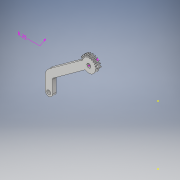
# Autodesk Inventor part: sem2_thumb-finger2
Saved by Autodesk Inventor 2018 (Build 220112000, 112)
## iProperties
Created: 2017-10-02
Part Number: sem2_thumb-finger2
Material: Generic
Document SubType Name: Modeling
Designer: rheal
Density: 1 g/cm^3
Appearance: Default
Author: rheal
Autodesk Inventor part; units mm, degrees
note: some values were not read from the file. Chosen so that the rebuilt part matches the saved one: pattern direction of "Circular Pattern2".
ref_plane "YZ Plane" through (0, 0, 0) normal (1, 0, 0) x (0, 1, 0)
ref_plane "XZ Plane" through (0, 0, 0) normal (0, 1, 0) x (-1, 0, 0)
ref_plane "XY Plane" through (0, 0, 0) normal (0, 0, 1) x (1, 0, 0)
sketch "Sketch1" plane through (0, 0, 0) normal (0, 0, 1) x (1, 0, 0)
  arc A0 (-83.5272, 11.9642) -> (-77.9867, 11.6439) centre (-80.7477, 11.9642) ccw
  line L0 (-50.0146, 32.1007) -> (-50.0146, 50.0136) construction
  arc A1 (-52.8662, 40.9092) -> (-54.8238, 46.3734) centre (-50.0146, 45.0136) ccw
  line L1 (-83.5272, 11.9642) -> (-83.5272, 22.4192)
  arc A2 (-83.5272, 11.9642) -> (-77.9681, 11.9642) centre (-80.7477, 11.9642) ccw
  line L2 (-77.9681, 11.9642) -> (-77.9681, 21.7768)
  line L3 (-52.8662, 40.9092) -> (-77.1364, 23.2751)
  line L4 (-80.4111, 27.7823) -> (-56.141, 45.4163)
  arc A3 (-80.4111, 27.7823) -> (-83.5272, 22.4192) centre (-76.1194, 21.702) ccw
  arc A4 (-77.1364, 23.2751) -> (-77.9681, 21.7768) centre (-76.2028, 21.7768) ccw
  line L5 (-52.8662, 40.9092) -> (-56.141, 45.4163)
  line L6 (-77.1364, 23.2751) -> (-80.4111, 27.7823)
  line L7 (-56.141, 45.4163) -> (-54.8238, 46.3734)
  arc A5 (-54.7992, 43.5696) -> (-54.8238, 46.3734) centre (-50.0146, 45.0136) ccw
  line L8 (-52.8662, 40.9092) -> (-77.1364, 23.2751)
  line L9 (-77.1364, 23.2751) -> (-80.4111, 27.7823)
  point P0 (19.05, 139.7)
  point P1 (-45.0223, 44.7358)
  point P2 (-77.9681, 22.6804)
  dimension "d69" = 2.7795
  dimension "d107" = 30
  constraints: 20 end point, 13 point on circle, 6 centre point, 2 perpendicular, 2 point on line, 2 tangent, 2 vertical, 1 coincident, 1 collinear, 1 concentric, 1 parallel
  measures "d69" radius of A0
  measures "d107" distance of L3.end L3.start
extrude "Extrusion1" add sketch "Sketch1" along normal blind 3
sketch "Sketch15" plane through (0, 0, 0) normal (0, 0, -1) x (-1, 0, 0)
  point P0 (0, 0)
sketch "Sketch16" plane through (0, 0, 0) normal (0, 0, -1) x (-1, 0, 0)
  circle A0 centre (50, 45) radius 2.5 projected
  line L0 (50, 45) -> (50, 42.5) construction
  line L1 (50, 45) -> (52.5, 45) construction
  point P0 (0, 0)
  constraints: 4 end point, 2 point on circle, 1 perpendicular, 1 vertical
ref_plane "Work Plane2" through (-50, 45, 0) normal (0, -1, 0) x (1, 0, 0)
sketch "Sketch18" plane through (-50, 45, 0) normal (0, -1, 0) x (1, 0, 0)
  line L0 (0, 0.0908) -> (0, 2.9092) construction
  line L1 (0, 1.5) -> (0, -3.9375) construction
  point P0 (50, 0)
  constraints: 2 end point, 1 midpoint, 1 vertical
sketch "Sketch19" plane through (0, 0, 0) normal (0, 0, -1) x (-1, 0, 0)
  line L0 (40.2723, 49.5) -> (49.7354, 49.2661) construction
  line L1 (49.9819, 50.3977) -> (49.9819, 51.6759) construction
  line L2 (49.9819, 49.9276) -> (49.4819, 49.9276)
  line L3 (49.7319, 51.6759) -> (49.7319, 50.8959)
  arc A0 (49.7319, 50.8959) -> (49.4819, 49.9276) centre (51.3636, 49.9582) ccw
  line L4 (49.7319, 51.6759) -> (49.9819, 51.6759)
  line L5 (59.7277, 49.5) -> (49.7354, 49.2661) construction
  line L6 (49.9819, 49.9276) -> (50.4819, 49.9276)
  line L7 (50.2319, 51.6759) -> (50.2319, 50.8959)
  arc A1 (50.4819, 49.9276) -> (50.2319, 50.8959) centre (48.6002, 49.9582) ccw
  line L8 (50.2319, 51.6759) -> (49.9819, 51.6759)
  point P0 (0, 0)
  point P1 (50, 50)
  dimension "d82" = 1.676
  dimension "d83" = 0.5
  dimension "d84" = 0.25
  dimension "d85" = 1
  dimension "d86" = 0.0746
  constraints: 18 end point, 4 point on circle, 4 symmetric about line, 2 centre point, 1 perpendicular, 1 vertical, 1 other
  measures "d82" distance of point (50, 50) L1.end
  measures "d83" distance of L2.start L2.end
  measures "d84" distance between parallel lines of L1 L3
  measures "d85" distance of L3.end L2.end
  measures "d86" distance of point (50, 50) L2.start
extrude "Extrusion13" add sketch "Sketch19" against normal blind 3
sketch "Sketch20" plane through (0, 0, 0) normal (0, 0, -1) x (-1, 0, 0)
  line L0 (45.7576, 49.2502) -> (46.1486, 48.8898) projected
  line L1 (46.9253, 49.5288) -> (46.647, 49.982) projected
  point P0 (0, 0)
sketch "Sketch21" plane through (0, 0, 0) normal (0, 0, -1) x (-1, 0, 0)
  arc A0 (49.5542, 49.9801) -> (46.9563, 41.0331) centre (50, 45) ccw projected
  circle A1 centre (50, 45) radius 1.5
  point P0 (0, 0)
  dimension "d94" = 3
  constraints: 1 centre point, 1 coincident
  measures "d94" diameter of A1
extrude "Extrusion15" cut sketch "Sketch21" against normal blind 3
pattern_circular "Circular Pattern2" count 10 over 142 about axis through (-50, 45, 0) along (0, 0, -1) of "Extrusion13" both ways yes
sketch "Sketch22" plane through (0, 0, 3) normal (0, 0, 1) x (1, 0, 0)
  arc A0 (-83.5272, 11.9642) -> (-77.9681, 11.9642) centre (-80.7477, 11.9642) ccw projected
  circle A1 centre (-80.7477, 11.9642) radius 1.5
  point P0 (0, 0)
  dimension "d108" = 3
  constraints: 1 centre point, 1 coincident
  measures "d108" diameter of A1
extrude "Extrusion16" cut sketch "Sketch22" against normal through all
body "Solid1"
